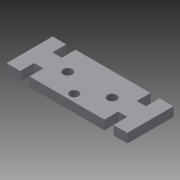
# Autodesk Inventor part: prepazka_2x_lozisko_1x_dira
Saved by Autodesk Inventor 2015 (Build 190159000, 159)
## iProperties
Created: 2012-08-25
Part Number: prepazka_2x_lozisko_1x_dira
Material: Generic
Document SubType Name: Modeling
Designer: idle-rug
Density: 1 g/cm^3
Appearance: Default
Author: idle-rug
Autodesk Inventor part; units mm, degrees
ref_plane "YZ Plane" through (0, 0, 0) normal (1, 0, 0) x (0, 1, 0)
ref_plane "XZ Plane" through (0, 0, 0) normal (0, 1, 0) x (-1, 0, 0)
sketch "Sketch1" plane through (0, 0, 0) normal (0, 0, 1) x (1, 0, 0)
  line L0 (65.5, 25) -> (-65.5, 25)
  line L1 (-65.5, 25) -> (-65.5, -25)
  line L2 (-65.5, -25) -> (65.5, -25)
  line L3 (65.5, -25) -> (65.5, 25)
  line L4 (-40.6, 25) -> (-40.6, 10)
  line L5 (-40.6, 10) -> (-50.6, 10)
  line L6 (-50.6, 10) -> (-50.6, 25)
  line L7 (-40.6, -25) -> (-40.6, -10)
  line L8 (-40.6, -10) -> (-50.6, -10)
  line L9 (-50.6, -10) -> (-50.6, -25)
  line L10 (40.6, 25) -> (40.6, 10)
  line L11 (40.6, 10) -> (50.6, 10)
  line L12 (50.6, 10) -> (50.6, 25)
  line L13 (40.6, -25) -> (40.6, -10)
  line L14 (40.6, -10) -> (50.6, -10)
  line L15 (50.6, -10) -> (50.6, -25)
  circle A0 centre (24.1, 0) radius 7.5
  circle A1 centre (-24.1, 0) radius 7.5
  line L16 (0, -25) -> (0, -17)
  circle A2 centre (0, -17) radius 4.75
  circle A3 centre (-24.1, 0) radius 5
  circle A4 centre (24.1, 0) radius 5
  point P0 (0, 0)
  point P1 (0, 0)
  dimension "d0" = 15
  dimension "d1" = 15
  dimension "d2" = 15
  dimension "d3" = 15
  dimension "d8" = 15
  dimension "d9" = 15
  dimension "d23" = 8
  dimension "d24" = 9.5
  dimension "d27" = 10
  dimension "d28" = 10
  constraints: 34 end point, 8 point on line, 7 perpendicular, 5 centre point, 3 coincident, 1 midpoint, 1 vertical
  measures "d0" distance of L4.start L4.end
  measures "d1" distance of L7.start L7.end
  measures "d2" distance of L10.start L10.end
  measures "d3" distance of L13.start L13.end
  measures "d8" diameter of A0
  measures "d9" diameter of A1
  measures "d23" distance of L16.start L16.end
  measures "d24" diameter of A2
  measures "d27" diameter of A3
  measures "d28" diameter of A4
ref_plane "Work Plane1" through (-40.6, 25, 0) normal (0, 1, 0) x (1, 0, 0)
sketch "Sketch2" plane through (-40.6, 25, 0) normal (0, 1, 0) x (1, 0, 0)
  circle A0 centre (40.6, -5) radius 1.25
  point P0 (40.6, 0)
  dimension "d20" = 2.5
  constraints: 1 centre point
  measures "d20" diameter of A0
extrude "Extrusion11" add sketch "Sketch1" along normal blind 10 contours L3 L2 L15 L14 L13 L7 L8 L9 L1 L0 L6 L5 L4 L10 L11 L12 | A0 | A1
extrude "Extrusion12" cut sketch "Sketch1" along normal blind 8 contours A0 | A1
sketch "Sketch4" plane through (-40.6, 25, 0) normal (0, 1, 0) x (1, 0, 0)
  line L0 (40.6, 0) -> (40.6, -5)
  circle A0 centre (40.6, -5) radius 1.25
  dimension "d50" = 5
  dimension "d51" = 2.5
  constraints: 2 end point, 1 centre point, 1 coincident, 1 vertical
  measures "d50" distance of L0.start L0.end
  measures "d51" diameter of A0
extrude "Extrusion14" cut sketch "Sketch4" against normal blind 10
fillet "Fillet1" radius 2 2 edges at (-31.6, 0, 0) (16.6, 0, 0)
body "Solid3"
